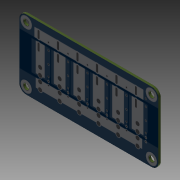
# Autodesk Inventor part: PCB
Saved by Autodesk Inventor 2014 SP1 (Build 180222100, 222)
## iProperties
Created: 2016-03-18
Part Number: PCB
Material: Generic
Document SubType Name: Modeling
Designer: Tyler
Density: 1 g/cm^3
Appearance: Dark Olive
Author: Tyler
Autodesk Inventor part; units mm, degrees
ref_plane "YZ Plane" through (0, 0, 0) normal (1, 0, 0) x (0, 1, 0)
ref_plane "XZ Plane" through (0, 0, 0) normal (0, 1, 0) x (-1, 0, 0)
ref_plane "XY Plane" through (0, 0, 0) normal (0, 0, 1) x (1, 0, 0)
sketch "Sketch1" plane through (0, 0, 0) normal (0, 1, 0) x (-1, 0, 0)
  line L0 (-50, -25) -> (50, -25)
  line L1 (50, -25) -> (50, 25)
  line L2 (50, 25) -> (-50, 25)
  line L3 (-50, 25) -> (-50, -25)
  line L4 (-50, -25) -> (50, 25) construction
  line L5 (50, -25) -> (-50, 25) construction
  point P0 (0, 0)
  dimension "d0" = 100
  dimension "d1" = 50
  constraints: 12 end point, 2 midpoint, 2 parallel, 1 horizontal, 1 perpendicular
  measures "d0" distance of L2.end L1.end
  measures "d1" distance of L1.end L0.end
extrude "Extrusion1" add sketch "Sketch1" along normal blind 1.6
fillet "Fillet1" radius 5 4 edges at (50, 0.8, 25) (-50, 0.8, 25) (-50, 0.8, -25) (50, 0.8, -25)
sketch "Sketch2" plane through (0, 1.6, 0) normal (0, 1, 0) x (1, 0, 0)
  arc A0 (50, 20) -> (45, 25) centre (45, 20) ccw projected
  arc A1 (-45, 25) -> (-50, 20) centre (-45, 20) ccw projected
  arc A2 (-50, -20) -> (-45, -25) centre (-45, -20) ccw projected
  arc A3 (45, -25) -> (50, -20) centre (45, -20) ccw projected
  point P0 (0, 0)
  constraints: 4 coincident
hole "Hole1" at (-45, 1.6, -20) at (-45, 1.6, 20) at (45, 1.6, 20) at (45, 1.6, -20) direction (0, -1, 0) diameter 4 end through all
body "Solid1"
